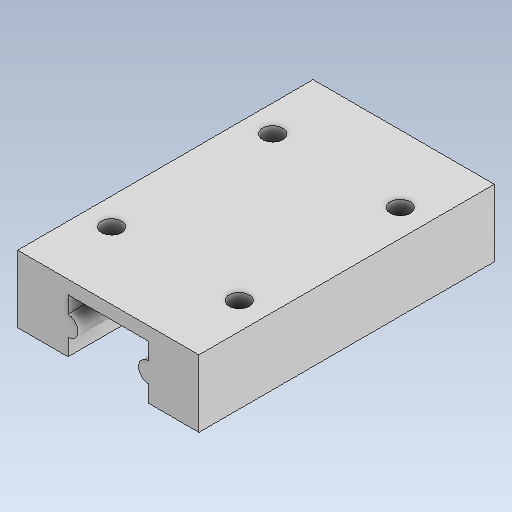
# Autodesk Inventor part: 滑轨座
Saved by Autodesk Inventor 2020 (Build 240168000, 168)
## iProperties
Created: 2020-12-02
Part Number: 滑轨座
Material: 常规
Document SubType Name: Sheet Metal
Designer: huang
Density: 1 g/cm^3
Sheet Metal Rule: 默认_mm
Appearance: 默认
Author: huang
Autodesk Inventor part; units mm, degrees
ref_plane "YZ Plane" through (0, 0, 0) normal (1, 0, 0) x (0, 1, 0)
ref_plane "XZ Plane" through (0, 0, 0) normal (0, 1, 0) x (-1, 0, 0)
ref_plane "XY Plane" through (0, 0, 0) normal (0, 0, 1) x (1, 0, 0)
sketch "草图1" plane through (0, 0, 0) normal (0, 1, 0) x (-1, 0, 0)
  line L0 (0, 0) -> (27, 0)
  line L1 (27, 0) -> (27, -44)
  line L2 (27, -44) -> (0, -44)
  line L3 (0, -44) -> (0, 0)
  dimension "d0" = 44
  dimension "d1" = 27
  constraints: 8 end point, 2 parallel, 1 horizontal, 1 perpendicular
  measures "d0" distance of L0.end L1.end
  measures "d1" distance of L1.end L2.end
extrude "拉伸1" add sketch "草图1" along normal blind 10
sketch "草图2" plane through (-27, 0, 0) normal (0, 0, 1) x (1, 0, 0)
  line L0 (0, 10) -> (27, 10) projected
  line L1 (13.5, 10) -> (13.5, 0)
  line L2 (13.5, 10) -> (7.5, 10)
  line L3 (7.5, 10) -> (19.5, 10)
  line L4 (7.5, 10) -> (7.5, 0)
  line L5 (0, 0) -> (27, 0) projected
  line L6 (19.5, 10) -> (19.5, 0)
  line L7 (7.5, 0) -> (19.5, 0)
  line L8 (7.5, 0) -> (19.5, 0)
  line L9 (19.5, 0) -> (19.5, 8)
  line L10 (19.5, 8) -> (7.5, 8)
  line L11 (7.5, 8) -> (7.5, 0)
  point P0 (7.5, 8)
  dimension "d19" = 6
  dimension "d20" = 12
  dimension "d21" = 8
  constraints: 20 end point, 5 point on line, 3 parallel, 2 perpendicular, 1 horizontal, 1 midpoint, 1 vertical
  measures "d19" distance of L1.start L2.end
  measures "d20" distance of L2.end L3.end
  measures "d21" distance between parallel lines of L5 L10
extrude "拉伸2" cut sketch "草图2" against normal through all contours L10 L1 L5 L4 | L10 L6 L5 L1
sketch "草图3" plane through (-27, 10, 0) normal (0, 0, 1) x (1, 0, 0)
  line L0 (7.5, -10) -> (7.5, -2) projected
  circle A0 centre (7.5, -6) radius 1.5
  line L1 (19.5, -2) -> (19.5, -10) projected
  circle A1 centre (19.5, -6) radius 1.5
  point P0 (27, -10)
  point P1 (19.5, -7.5)
  point P2 (19.5, -4.5)
  point P3 (7.5, -4.5)
  point P4 (7.5, -7.5)
  dimension "d22" = 3
  dimension "d23" = 3
  constraints: 2 centre point, 2 midpoint
  measures "d22" diameter of A0
  measures "d23" diameter of A1
extrude "拉伸3" add sketch "草图3" against normal blind 44 contours L0 A0 | L1 A1 picked at (8.2992, -6.2203) picked at (19.2676, -6.4427)
sketch "草图4" plane through (0, 10, 0) normal (0, 1, 0) x (1, 0, 0)
  circle A0 centre (-23, 34) radius 1.5
  line L0 (-6, 44) -> (-21, 44) projected
  circle A1 centre (-4, 34) radius 1.5
  circle A2 centre (-23, 10) radius 1.5
  circle A3 centre (-4, 10) radius 1.5
  line L1 (-27.606, 22) -> (3.9148, 22)
  line L2 (-13.5, 45.1542) -> (-13.5, -11.9454)
  point P0 (0, 0)
  point P1 (-27, 44)
  dimension "d15" = 3
  dimension "d24" = 12
  dimension "d25" = 9.5
  constraints: 4 centre point, 4 end point, 1 horizontal, 1 vertical
  measures "d15" diameter of A0
  measures "d24" distance from line of L1 A0.centre
  measures "d25" distance from line of L2 A0.centre
extrude "拉伸4" cut sketch "草图4" against normal blind 10
equation "\"折弯半径\" = 厚度"
equation "\"折弯释压宽度\" = 厚度"
equation "\"折弯释压深度\" = 0.5 * 厚度"
equation "\"拐角释压尺寸\" = 4 * 厚度"
equation "\"最小余量\" = 2 * 厚度"
equation "\"过渡半径\" = 折弯半径"
equation "\"Jacobi半径尺寸\" = 折弯半径"
equation "\"间隙大小\" = 厚度"
equation "\"厚度\" = 0.5"
